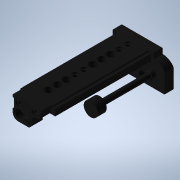
# Autodesk Inventor part: DGSL-12---(50-0-JP)
Saved by Autodesk Inventor 2021 (Build 250183000, 183)
## iProperties
Created: 2026-04-25
Part Number: DGSL-12---(50-0-JP)
Material: Generic
Catalog Web Link: www.3dfindit.com
Description: DGSL-(JP)-Plate
Vendor: FESTO
Document SubType Name: Modeling
Designer: psAdmin
Manufacturer: FESTO
Mass: 64.512 g
Surface Area: 242.987 cm^2
Volume: 64.512 cm^3
Density: 1 g/cm^3
Appearance: PSOLRGB-128-128-128
Category: PARTsolutions
Company: FESTO
Title: DGSL-12---(50-0-JP)
Author: Cadenas PARTsolutions
Comments: Plate
PSOL_IDENT_0: {$CADENAS_DATA/23d-libs/festo/parts/d/dgsl/parts/dgsl_jochplatten.prj},193 {VTYP=3D},{NB=DGSL-12---(
PSOL_IDENT_1: 50-0-JP)},{LINA=DGSL-12---(50-0-JP)},{NN=DGSL-(JP)},{DATE=08.01.2026 09:08:18},{GEOMDATE=08.01.2026
PSOL_IDENT_2: 09:08:00},{VERSION=},{LINEID=50},{WBVAR=DA,HUB},{WBNUMERIC=DA,HUB}  {NB=DGSL-12---(50-0-JP)},{LINA=D
PSOL_IDENT_3: GSL-12---(50-0-JP)},{KT=DUMMY},{TYP=DGSL-12},{KDM2=12},{DA=0},{HUB=50},{L1=108.6},{L1X=230.000},{SDD
PSOL_IDENT_4: N=10.000},{YOFF=0.000},{HUBW=[10:200]},{L2=10.000},{L4=50.000},{L9=10.000},{L15=5.800},{B4=24.000},{
PSOL_IDENT_5: B5=10.000},{BM=23.500},{H2=34.800},{H11=10.000},{H12=17.700},{KDM=16},{DIMBOHR=23.500},{DIMBOHRY=-15
PSOL_IDENT_6: .800},{KORRB4=0.200},{KORRH12=0.000},{A=1.750}
NB: DGSL-12---(50-0-JP)
NN: DGSL-(JP)
NT: Plate
NBSYN: $TYP.---($HUB.-$DA.-JP)
LINA: DGSL-12---(50-0-JP)
CATALOG: Festo
TYP: DGSL-12
KDM2: 12
DA: 0
HUB: 50
YOFF: 0
HUBW: [10:200]
L2: 10
L4: 50
L9: 10
L15: 5.8
B4: 24
B5: 10
BM: 23.5
H2: 34.8
H11: 10
H12: 17.7
KDM: 16
DIMBOHR: 23.5
DIMBOHRY: -15.8
KORRB4: 0.2
KORRH12: 0
A: 1.75
SUPPLIER: FESTO
ARTICLENO: DGSL-12---(50-0-JP)
BOMINFO: DGSL-12---(50-0-JP)
CREATOR: CADENAS GmbH
Autodesk Inventor part; units mm, degrees
sketch "Skizze_Jochplatte" plane through (0, 0, 0) normal (0, 0, 1) x (1, 0, 0)
  line L0 (0, 34.3) -> (0, 0)
  line L1 (0, 0) -> (58.5, 0)
  arc A0 (58.5, 0) -> (59, 0.5) centre (58.5, 0.5) ccw
  line L2 (59, 0.5) -> (59, 21.9765)
  arc A1 (59, 21.9765) -> (58.814286, 22.556964) centre (58, 21.9765) ccw
  arc A2 (58.814286, 22.556964) -> (46.894118, 28.847116) centre (46.6, 13.85) ccw
  arc A3 (46.6, 29.147059) -> (46.894118, 28.847116) centre (46.9, 29.147059) ccw
  line L3 (46.6, 29.147059) -> (46.6, 34.3)
  arc A4 (46.6, 34.3) -> (46.1, 34.8) centre (46.1, 34.3) ccw
  line L4 (46.1, 34.8) -> (0.5, 34.8)
  arc A5 (0.5, 34.8) -> (0, 34.3) centre (0.5, 34.3) ccw
  constraints: 12 point on circle, 10 end point, 6 centre point
sketch "Skizze_Jochplatte outline for Extrusion1" plane through (0, 0, 0) normal (0, 0, 1) x (1, 0, 0)
  arc A0 (0.5, 34.8) -> (0, 34.3) centre (0.5, 34.3) ccw
  line L0 (46.1, 34.8) -> (0.5, 34.8)
  arc A1 (46.6, 34.3) -> (46.1, 34.8) centre (46.1, 34.3) ccw
  line L1 (46.6, 29.147059) -> (46.6, 34.3)
  arc A2 (46.894118, 28.847116) -> (46.6, 29.147059) centre (46.9, 29.147059) cw
  arc A3 (58.814286, 22.556964) -> (46.894118, 28.847116) centre (46.6, 13.85) ccw
  arc A4 (59, 21.9765) -> (58.814286, 22.556964) centre (58, 21.9765) ccw
  line L2 (59, 0.5) -> (59, 21.9765)
  arc A5 (58.5, 0) -> (59, 0.5) centre (58.5, 0.5) ccw
  line L3 (0, 0) -> (58.5, 0)
  line L4 (0, 34.3) -> (0, 0)
extrude "Extrusion1" add sketch "Skizze_Jochplatte outline for Extrusion1" along normal blind 10
sketch "Sketch2" plane through (0, 0, 0) normal (0, 0, -1) x (-1, 0, 0)
  point P0 (-13.5, 7.1)
hole "Hole1" at (13.5, 7.1, 0) direction (0, 0, 1) diameter 7.8 depth 10 counterbore diameter 8 counterbore depth 7.5
sketch "Sketch3" plane through (0, 0, 0) normal (0, 0, -1) x (-1, 0, 0)
  point P0 (-33.5, 7.1)
hole "Hole2" at (33.5, 7.1, 0) direction (0, 0, 1) diameter 7.8 depth 10 counterbore diameter 8 counterbore depth 7.5
sketch "Skizze_JP_Bohrung_1C" plane through (0, 7.1, 0) normal (0, 1, 0) x (1, 0, 0)
  line L0 (23.5, -10) -> (23.5, 0)
  line L1 (23.5, 0) -> (27, 0)
  line L2 (27, 0) -> (27, -1.6)
  line L3 (27, -1.6) -> (26, -1.6)
  line L4 (26, -1.6) -> (25.567, -2.033)
  line L5 (25.567, -2.033) -> (25.567, -9.567)
  line L6 (25.567, -9.567) -> (26, -10)
  line L7 (26, -10) -> (23.5, -10)
  line L8 (23.5, -10) -> (23.5, 0)
  constraints: 18 end point
sketch "Skizze_JP_Bohrung_1C outline for Revolution1" plane through (0, 7.1, 0) normal (0, 1, 0) x (1, 0, 0)
  line L0 (23.5, 0) -> (27, 0)
  line L1 (27, 0) -> (27, -1.6)
  line L2 (27, -1.6) -> (26, -1.6)
  line L3 (26, -1.6) -> (25.567, -2.033)
  line L4 (25.567, -2.033) -> (25.567, -9.567)
  line L5 (25.567, -9.567) -> (26, -10)
  line L6 (26, -10) -> (23.5, -10)
  line L7 (23.5, -10) -> (23.5, 0)
revolve "Revolution1" cut sketch "Skizze_JP_Bohrung_1C outline for Revolution1" angle 360 about axis through (23.5, 7.1, 10) along (0, 0, 1)
thread "Thread1" size "M5x0.8" class "6H" standard "ISO Metric profile" full length
sketch "Skizze_JP_Bohrung_2A" plane through (0, 17.1, 0) normal (0, 1, 0) x (1, 0, 0)
  line L0 (13.5, -10) -> (13.5, 0)
  line L1 (13.5, 0) -> (17, 0)
  line L2 (17, 0) -> (17, -1.6)
  line L3 (17, -1.6) -> (16, -1.6)
  line L4 (16, -1.6) -> (15.567, -2.033)
  line L5 (15.567, -2.033) -> (15.567, -9.567)
  line L6 (15.567, -9.567) -> (16, -10)
  line L7 (16, -10) -> (13.5, -10)
  line L8 (13.5, -10) -> (13.5, 0)
  constraints: 18 end point
sketch "Skizze_JP_Bohrung_2A outline for Revolution2" plane through (0, 17.1, 0) normal (0, 1, 0) x (1, 0, 0)
  line L0 (13.5, 0) -> (17, 0)
  line L1 (17, 0) -> (17, -1.6)
  line L2 (17, -1.6) -> (16, -1.6)
  line L3 (16, -1.6) -> (15.567, -2.033)
  line L4 (15.567, -2.033) -> (15.567, -9.567)
  line L5 (15.567, -9.567) -> (16, -10)
  line L6 (16, -10) -> (13.5, -10)
  line L7 (13.5, -10) -> (13.5, 0)
revolve "Revolution2" cut sketch "Skizze_JP_Bohrung_2A outline for Revolution2" angle 360 about axis through (13.5, 17.1, 10) along (0, 0, 1)
thread "Thread2" size "M5x0.8" class "6H" standard "ISO Metric profile" full length
sketch "Skizze_JP_Bohrung_2B" plane through (0, 17.1, 0) normal (0, 1, 0) x (1, 0, 0)
  line L0 (23.5, -10) -> (23.5, 0)
  line L1 (23.5, 0) -> (27, 0)
  line L2 (27, 0) -> (27, -1.6)
  line L3 (27, -1.6) -> (26, -1.6)
  line L4 (26, -1.6) -> (25.567, -2.033)
  line L5 (25.567, -2.033) -> (25.567, -9.567)
  line L6 (25.567, -9.567) -> (26, -10)
  line L7 (26, -10) -> (23.5, -10)
  line L8 (23.5, -10) -> (23.5, 0)
  constraints: 18 end point
sketch "Skizze_JP_Bohrung_2B outline for Revolution3" plane through (0, 17.1, 0) normal (0, 1, 0) x (1, 0, 0)
  line L0 (23.5, 0) -> (27, 0)
  line L1 (27, 0) -> (27, -1.6)
  line L2 (27, -1.6) -> (26, -1.6)
  line L3 (26, -1.6) -> (25.567, -2.033)
  line L4 (25.567, -2.033) -> (25.567, -9.567)
  line L5 (25.567, -9.567) -> (26, -10)
  line L6 (26, -10) -> (23.5, -10)
  line L7 (23.5, -10) -> (23.5, 0)
revolve "Revolution3" cut sketch "Skizze_JP_Bohrung_2B outline for Revolution3" angle 360 about axis through (23.5, 17.1, 10) along (0, 0, 1)
thread "Thread3" size "M5x0.8" class "6H" standard "ISO Metric profile" full length
sketch "Skizze_JP_Bohrung_2C" plane through (0, 17.1, 0) normal (0, 1, 0) x (1, 0, 0)
  line L0 (33.5, -10) -> (33.5, 0)
  line L1 (33.5, 0) -> (37, 0)
  line L2 (37, 0) -> (37, -1.6)
  line L3 (37, -1.6) -> (36, -1.6)
  line L4 (36, -1.6) -> (35.567, -2.033)
  line L5 (35.567, -2.033) -> (35.567, -9.567)
  line L6 (35.567, -9.567) -> (36, -10)
  line L7 (36, -10) -> (33.5, -10)
  line L8 (33.5, -10) -> (33.5, 0)
  constraints: 18 end point
sketch "Skizze_JP_Bohrung_2C outline for Revolution4" plane through (0, 17.1, 0) normal (0, 1, 0) x (1, 0, 0)
  line L0 (33.5, 0) -> (37, 0)
  line L1 (37, 0) -> (37, -1.6)
  line L2 (37, -1.6) -> (36, -1.6)
  line L3 (36, -1.6) -> (35.567, -2.033)
  line L4 (35.567, -2.033) -> (35.567, -9.567)
  line L5 (35.567, -9.567) -> (36, -10)
  line L6 (36, -10) -> (33.5, -10)
  line L7 (33.5, -10) -> (33.5, 0)
revolve "Revolution4" cut sketch "Skizze_JP_Bohrung_2C outline for Revolution4" angle 360 about axis through (33.5, 17.1, 10) along (0, 0, 1)
thread "Thread4" size "M5x0.8" class "6H" standard "ISO Metric profile" full length
sketch "Skizze_JP_Bohrung_3" plane through (0, 27.1, 0) normal (0, 1, 0) x (1, 0, 0)
  line L0 (23.5, -10) -> (23.5, 0)
  line L1 (23.5, 0) -> (27, 0)
  line L2 (27, 0) -> (27, -1.6)
  line L3 (27, -1.6) -> (26, -1.6)
  line L4 (26, -1.6) -> (25.567, -2.033)
  line L5 (25.567, -2.033) -> (25.567, -9.567)
  line L6 (25.567, -9.567) -> (26, -10)
  line L7 (26, -10) -> (23.5, -10)
  line L8 (23.5, -10) -> (23.5, 0)
  constraints: 18 end point
sketch "Skizze_JP_Bohrung_3 outline for Revolution5" plane through (0, 27.1, 0) normal (0, 1, 0) x (1, 0, 0)
  line L0 (23.5, 0) -> (27, 0)
  line L1 (27, 0) -> (27, -1.6)
  line L2 (27, -1.6) -> (26, -1.6)
  line L3 (26, -1.6) -> (25.567, -2.033)
  line L4 (25.567, -2.033) -> (25.567, -9.567)
  line L5 (25.567, -9.567) -> (26, -10)
  line L6 (26, -10) -> (23.5, -10)
  line L7 (23.5, -10) -> (23.5, 0)
revolve "Revolution5" cut sketch "Skizze_JP_Bohrung_3 outline for Revolution5" angle 360 about axis through (23.5, 27.1, 10) along (0, 0, 1)
thread "Thread5" size "M5x0.8" class "6H" standard "ISO Metric profile" full length
sketch "Sketch_2" plane through (0, 29.6, 0) normal (0, 1, 0) x (1, 0, 0)
  line L0 (14.5, -4.6) -> (14.5, 0)
  line L1 (14.5, 0) -> (18.5, 0)
  line L2 (18.5, 0) -> (18.5, -4.6)
  line L3 (18.5, -4.6) -> (18.45, -4.6)
  line L4 (18.45, -4.6) -> (18.45, -1)
  arc A0 (18.45, -1) -> (18.05, -0.6) centre (18.05, -1) ccw
  line L5 (18.05, -0.6) -> (14.5, -0.6)
  line L6 (14.5, -0.6) -> (14.5, 0)
  constraints: 14 end point, 2 point on circle, 1 centre point
sketch "Sketch_2 outline for Revolution6" plane through (0, 29.6, 0) normal (0, 1, 0) x (1, 0, 0)
  line L0 (14.5, 0) -> (18.5, 0)
  line L1 (18.5, 0) -> (18.5, -4.6)
  line L2 (18.5, -4.6) -> (18.45, -4.6)
  line L3 (18.45, -4.6) -> (18.45, -1)
  arc A0 (18.45, -1) -> (18.05, -0.6) centre (18.05, -1) ccw
  line L4 (18.05, -0.6) -> (14.5, -0.6)
  line L5 (14.5, -0.6) -> (14.5, 0)
revolve "Revolution6" cut sketch "Sketch_2 outline for Revolution6" angle 360 about axis through (14.5, 29.6, 4.6) along (0, 0, 1)
sketch "Sketch_8" plane through (0, 29.6, 0) normal (0, 1, 0) x (1, 0, 0)
  line L0 (32.5, -4.6) -> (32.5, 0)
  line L1 (32.5, 0) -> (36.5, 0)
  line L2 (36.5, 0) -> (36.5, -4.6)
  line L3 (36.5, -4.6) -> (36.45, -4.6)
  line L4 (36.45, -4.6) -> (36.45, -1)
  arc A0 (36.45, -1) -> (36.05, -0.6) centre (36.05, -1) ccw
  line L5 (36.05, -0.6) -> (32.5, -0.6)
  line L6 (32.5, -0.6) -> (32.5, 0)
  constraints: 14 end point, 2 point on circle, 1 centre point
sketch "Sketch_8 outline for Revolution7" plane through (0, 29.6, 0) normal (0, 1, 0) x (1, 0, 0)
  line L0 (32.5, 0) -> (36.5, 0)
  line L1 (36.5, 0) -> (36.5, -4.6)
  line L2 (36.5, -4.6) -> (36.45, -4.6)
  line L3 (36.45, -4.6) -> (36.45, -1)
  arc A0 (36.45, -1) -> (36.05, -0.6) centre (36.05, -1) ccw
  line L4 (36.05, -0.6) -> (32.5, -0.6)
  line L5 (32.5, -0.6) -> (32.5, 0)
revolve "Revolution7" cut sketch "Sketch_8 outline for Revolution7" angle 360 about axis through (32.5, 29.6, 4.6) along (0, 0, 1)
sketch "Sketch_7" plane through (14.5, 29.6, 0.6) normal (0, 0, -1) x (1, 0, 0)
  line L0 (-1.5, -0.866025) -> (0, -1.732051)
  line L1 (0, -1.732051) -> (1.5, -0.866025)
  line L2 (1.5, -0.866025) -> (1.5, 0.866025)
  line L3 (1.5, 0.866025) -> (0, 1.732051)
  line L4 (0, 1.732051) -> (-1.5, 0.866025)
  line L5 (-1.5, 0.866025) -> (-1.5, -0.866025)
  constraints: 12 end point
sketch "Sketch_7 outline for Extrusion2" plane through (14.5, 29.6, 0.6) normal (0, 0, -1) x (1, 0, 0)
  line L0 (-1.5, 0.866025) -> (-1.5, -0.866025)
  line L1 (0, 1.732051) -> (-1.5, 0.866025)
  line L2 (1.5, 0.866025) -> (0, 1.732051)
  line L3 (1.5, -0.866025) -> (1.5, 0.866025)
  line L4 (0, -1.732051) -> (1.5, -0.866025)
  line L5 (-1.5, -0.866025) -> (0, -1.732051)
extrude "Extrusion2" cut sketch "Sketch_7 outline for Extrusion2" against normal blind 2.2
sketch "Sketch_15" plane through (32.5, 29.6, 0.6) normal (0, 0, -1) x (1, 0, 0)
  line L0 (-1.5, -0.866025) -> (0, -1.732051)
  line L1 (0, -1.732051) -> (1.5, -0.866025)
  line L2 (1.5, -0.866025) -> (1.5, 0.866025)
  line L3 (1.5, 0.866025) -> (0, 1.732051)
  line L4 (0, 1.732051) -> (-1.5, 0.866025)
  line L5 (-1.5, 0.866025) -> (-1.5, -0.866025)
  constraints: 12 end point
sketch "Sketch_15 outline for Extrusion3" plane through (32.5, 29.6, 0.6) normal (0, 0, -1) x (1, 0, 0)
  line L0 (-1.5, 0.866025) -> (-1.5, -0.866025)
  line L1 (0, 1.732051) -> (-1.5, 0.866025)
  line L2 (1.5, 0.866025) -> (0, 1.732051)
  line L3 (1.5, -0.866025) -> (1.5, 0.866025)
  line L4 (0, -1.732051) -> (1.5, -0.866025)
  line L5 (-1.5, -0.866025) -> (0, -1.732051)
extrude "Extrusion3" cut sketch "Sketch_15 outline for Extrusion3" against normal blind 2.2
sketch "Skizze_JP_Bohrung_5" plane through (0, 13.8, 0) normal (0, 1, 0) x (1, 0, 0)
  line L0 (45.1, -4.6) -> (45.1, 0)
  line L1 (45.1, 0) -> (49.1, 0)
  line L2 (49.1, 0) -> (49.1, -4.6)
  line L3 (49.1, -4.6) -> (48.6, -4.6)
  line L4 (48.6, -4.6) -> (48.6, -1)
  arc A0 (48.6, -1) -> (48.2, -0.6) centre (48.2, -1) ccw
  line L5 (48.2, -0.6) -> (46.842, -0.6)
  line L6 (46.842, -0.6) -> (45.1, -1.234036)
  line L7 (45.1, -1.234036) -> (45.1, 0)
  constraints: 16 end point, 2 point on circle, 1 centre point
sketch "Skizze_JP_Bohrung_5 outline for Revolution8" plane through (0, 13.8, 0) normal (0, 1, 0) x (1, 0, 0)
  line L0 (45.1, 0) -> (49.1, 0)
  line L1 (49.1, 0) -> (49.1, -4.6)
  line L2 (49.1, -4.6) -> (48.6, -4.6)
  line L3 (48.6, -4.6) -> (48.6, -1)
  arc A0 (48.6, -1) -> (48.2, -0.6) centre (48.2, -1) ccw
  line L4 (48.2, -0.6) -> (46.842, -0.6)
  line L5 (46.842, -0.6) -> (45.1, -1.234036)
  line L6 (45.1, -1.234036) -> (45.1, 0)
revolve "Revolution8" cut sketch "Skizze_JP_Bohrung_5 outline for Revolution8" angle 360 about axis through (45.1, 13.8, 4.6) along (0, 0, 1)
sketch "Skizze_JP_Bohrung_5_HEX" plane through (45.1, 13.8, 0.6) normal (0, 0, -1) x (1, 0, 0)
  line L0 (-1.5, -0.866025) -> (0, -1.732051)
  line L1 (0, -1.732051) -> (1.5, -0.866025)
  line L2 (1.5, -0.866025) -> (1.5, 0.866025)
  line L3 (1.5, 0.866025) -> (0, 1.732051)
  line L4 (0, 1.732051) -> (-1.5, 0.866025)
  line L5 (-1.5, 0.866025) -> (-1.5, -0.866025)
  constraints: 12 end point
sketch "Skizze_JP_Bohrung_5_HEX outline for Extrusion4" plane through (45.1, 13.8, 0.6) normal (0, 0, -1) x (1, 0, 0)
  line L0 (-1.5, 0.866025) -> (-1.5, -0.866025)
  line L1 (0, 1.732051) -> (-1.5, 0.866025)
  line L2 (1.5, 0.866025) -> (0, 1.732051)
  line L3 (1.5, -0.866025) -> (1.5, 0.866025)
  line L4 (0, -1.732051) -> (1.5, -0.866025)
  line L5 (-1.5, -0.866025) -> (0, -1.732051)
extrude "Extrusion4" cut sketch "Skizze_JP_Bohrung_5_HEX outline for Extrusion4" against normal blind 2
sketch "Sketch_6" plane through (0, 13.8, 0) normal (0, 1, 0) x (1, 0, 0)
  line L0 (45.1, -80) -> (45.1, -10)
  line L1 (45.1, -10) -> (49.14, -10)
  line L2 (49.14, -10) -> (49.14, -14.15)
  line L3 (49.14, -14.15) -> (48.84, -14.45)
  line L4 (48.84, -14.45) -> (48.1, -14.45)
  line L5 (48.1, -14.45) -> (48.1, -70)
  line L6 (48.1, -70) -> (53.1, -70)
  line L7 (53.1, -70) -> (53.1, -80)
  line L8 (53.1, -80) -> (45.1, -80)
  line L9 (45.1, -80) -> (45.1, -10)
  constraints: 20 end point
sketch "Sketch_6 outline for Revolution9" plane through (0, 13.8, 0) normal (0, 1, 0) x (1, 0, 0)
  line L0 (45.1, -10) -> (49.14, -10)
  line L1 (49.14, -10) -> (49.14, -14.15)
  line L2 (49.14, -14.15) -> (48.84, -14.45)
  line L3 (48.84, -14.45) -> (48.1, -14.45)
  line L4 (48.1, -14.45) -> (48.1, -70)
  line L5 (48.1, -70) -> (53.1, -70)
  line L6 (53.1, -70) -> (53.1, -80)
  line L7 (53.1, -80) -> (45.1, -80)
  line L8 (45.1, -80) -> (45.1, -10)
revolve "Revolution9" add sketch "Sketch_6 outline for Revolution9" angle 360 about axis through (45.1, 13.8, 80) along (0, 0, 1)
sketch "Skizze_Schiene" plane through (0, 0, 10) normal (0, 0, 1) x (1, 0, 0)
  arc A0 (3.55, 25.3) -> (3.75, 25.1) centre (3.75, 25.3) ccw
  line L0 (3.75, 25.1) -> (11, 25.1)
  line L1 (11, 25.1) -> (11, 25)
  line L2 (11, 25) -> (36, 25)
  line L3 (36, 25) -> (36, 25.1)
  line L4 (36, 25.1) -> (43.25, 25.1)
  arc A1 (43.25, 25.1) -> (43.45, 25.3) centre (43.25, 25.3) ccw
  line L5 (43.45, 25.3) -> (43.45, 32.5)
  line L6 (43.45, 32.5) -> (40.5, 32.5)
  line L7 (40.5, 32.5) -> (40.5, 34.15359)
  line L8 (40.5, 34.15359) -> (41.1, 34.5)
  line L9 (41.1, 34.5) -> (41.1, 35)
  line L10 (41.1, 35) -> (5.9, 35)
  line L11 (5.9, 35) -> (5.9, 34.5)
  line L12 (5.9, 34.5) -> (6.5, 34.15359)
  line L13 (6.5, 34.15359) -> (6.5, 32.5)
  line L14 (6.5, 32.5) -> (3.55, 32.5)
  line L15 (3.55, 32.5) -> (3.55, 25.3)
  constraints: 32 end point, 4 point on circle, 2 centre point
sketch "Skizze_Schiene outline for Extrusion5" plane through (0, 0, 10) normal (0, 0, 1) x (1, 0, 0)
  line L0 (3.55, 32.5) -> (3.55, 25.3)
  line L1 (6.5, 32.5) -> (3.55, 32.5)
  line L2 (6.5, 34.15359) -> (6.5, 32.5)
  line L3 (5.9, 34.5) -> (6.5, 34.15359)
  line L4 (5.9, 35) -> (5.9, 34.5)
  line L5 (41.1, 35) -> (5.9, 35)
  line L6 (41.1, 34.5) -> (41.1, 35)
  line L7 (40.5, 34.15359) -> (41.1, 34.5)
  line L8 (40.5, 32.5) -> (40.5, 34.15359)
  line L9 (43.45, 32.5) -> (40.5, 32.5)
  line L10 (43.45, 25.3) -> (43.45, 32.5)
  arc A0 (43.25, 25.1) -> (43.45, 25.3) centre (43.25, 25.3) ccw
  line L11 (36, 25.1) -> (43.25, 25.1)
  line L12 (36, 25) -> (36, 25.1)
  line L13 (11, 25) -> (36, 25)
  line L14 (11, 25.1) -> (11, 25)
  line L15 (3.75, 25.1) -> (11, 25.1)
  arc A1 (3.55, 25.3) -> (3.75, 25.1) centre (3.75, 25.3) ccw
extrude "Extrusion5" add sketch "Skizze_Schiene outline for Extrusion5" along normal blind 108.6
sketch "Skizze_Endplatte" plane through (0, 0, 118.6) normal (0, 0, 1) x (1, 0, 0)
  line L0 (7.1, 32.65) -> (8.45, 31.3)
  line L1 (8.45, 31.3) -> (8.45, 22.5)
  line L2 (8.45, 22.5) -> (7.1, 21.15)
  line L3 (7.1, 21.15) -> (7.1, 17.2)
  arc A0 (7.1, 17.2) -> (13.1, 11.2) centre (13.1, 17.2) ccw
  line L4 (13.1, 11.2) -> (25.7, 11.2)
  line L5 (25.7, 11.2) -> (29.2, 14.7)
  line L6 (29.2, 14.7) -> (29.2, 21.5)
  arc A1 (32.2, 24.5) -> (29.2, 21.5) centre (32.2, 21.5) ccw
  line L7 (32.2, 24.5) -> (36.55, 24.5)
  line L8 (36.55, 24.5) -> (38.55, 26.5)
  line L9 (38.55, 26.5) -> (38.55, 31.3)
  line L10 (38.55, 31.3) -> (39.9, 32.65)
  line L11 (39.9, 32.65) -> (39.9, 34.8)
  line L12 (39.9, 34.8) -> (7.1, 34.8)
  line L13 (7.1, 34.8) -> (7.1, 32.65)
  constraints: 28 end point, 4 point on circle, 2 centre point
sketch "Skizze_Endplatte outline for Extrusion6" plane through (0, 0, 118.6) normal (0, 0, 1) x (1, 0, 0)
  line L0 (7.1, 34.8) -> (7.1, 32.65)
  line L1 (39.9, 34.8) -> (7.1, 34.8)
  line L2 (39.9, 32.65) -> (39.9, 34.8)
  line L3 (38.55, 31.3) -> (39.9, 32.65)
  line L4 (38.55, 26.5) -> (38.55, 31.3)
  line L5 (36.55, 24.5) -> (38.55, 26.5)
  line L6 (32.2, 24.5) -> (36.55, 24.5)
  arc A0 (29.2, 21.5) -> (32.2, 24.5) centre (32.2, 21.5) cw
  line L7 (29.2, 14.7) -> (29.2, 21.5)
  line L8 (25.7, 11.2) -> (29.2, 14.7)
  line L9 (13.1, 11.2) -> (25.7, 11.2)
  arc A1 (7.1, 17.2) -> (13.1, 11.2) centre (13.1, 17.2) ccw
  line L10 (7.1, 21.15) -> (7.1, 17.2)
  line L11 (8.45, 22.5) -> (7.1, 21.15)
  line L12 (8.45, 31.3) -> (8.45, 22.5)
  line L13 (7.1, 32.65) -> (8.45, 31.3)
extrude "Extrusion6" add sketch "Skizze_Endplatte outline for Extrusion6" along normal blind 12
sketch "Sketch_11" plane through (0, 29.6, 0) normal (0, 1, 0) x (1, 0, 0)
  line L0 (14.5, -130.6) -> (14.5, -126)
  line L1 (14.5, -130) -> (17.6, -130)
  arc A0 (17.6, -130) -> (18, -129.6) centre (17.6, -129.6) ccw
  line L2 (18, -129.6) -> (18, -126)
  line L3 (18, -126) -> (18.5, -126)
  line L4 (18.5, -126) -> (18.5, -130.6)
  line L5 (18.5, -130.6) -> (14.5, -130.6)
  line L6 (14.5, -130.6) -> (14.5, -130)
  constraints: 14 end point, 2 point on circle, 1 centre point
sketch "Sketch_11 outline for Revolution10" plane through (0, 29.6, 0) normal (0, 1, 0) x (1, 0, 0)
  line L0 (14.5, -130) -> (17.6, -130)
  arc A0 (17.6, -130) -> (18, -129.6) centre (17.6, -129.6) ccw
  line L1 (18, -129.6) -> (18, -126)
  line L2 (18, -126) -> (18.5, -126)
  line L3 (18.5, -126) -> (18.5, -130.6)
  line L4 (18.5, -130.6) -> (14.5, -130.6)
  line L5 (14.5, -130.6) -> (14.5, -130)
revolve "Revolution10" cut sketch "Sketch_11 outline for Revolution10" angle 360 about axis through (14.5, 29.6, 130.6) along (0, 0, 1)
sketch "Sketch_12" plane through (0, 29.6, 0) normal (0, 1, 0) x (1, 0, 0)
  line L0 (32.5, -130.6) -> (32.5, -126)
  line L1 (32.5, -130) -> (35.6, -130)
  arc A0 (35.6, -130) -> (36, -129.6) centre (35.6, -129.6) ccw
  line L2 (36, -129.6) -> (36, -126)
  line L3 (36, -126) -> (36.5, -126)
  line L4 (36.5, -126) -> (36.5, -130.6)
  line L5 (36.5, -130.6) -> (32.5, -130.6)
  line L6 (32.5, -130.6) -> (32.5, -130)
  constraints: 14 end point, 2 point on circle, 1 centre point
sketch "Sketch_12 outline for Revolution11" plane through (0, 29.6, 0) normal (0, 1, 0) x (1, 0, 0)
  line L0 (32.5, -130) -> (35.6, -130)
  arc A0 (35.6, -130) -> (36, -129.6) centre (35.6, -129.6) ccw
  line L1 (36, -129.6) -> (36, -126)
  line L2 (36, -126) -> (36.5, -126)
  line L3 (36.5, -126) -> (36.5, -130.6)
  line L4 (36.5, -130.6) -> (32.5, -130.6)
  line L5 (32.5, -130.6) -> (32.5, -130)
revolve "Revolution11" cut sketch "Sketch_12 outline for Revolution11" angle 360 about axis through (32.5, 29.6, 130.6) along (0, 0, 1)
sketch "Sketch_16" plane through (32.5, 29.6, 130) normal (0, 0, 1) x (1, 0, 0)
  line L0 (-1.732051, 0) -> (-0.866025, -1.5)
  line L1 (-0.866025, -1.5) -> (0.866025, -1.5)
  line L2 (0.866025, -1.5) -> (1.732051, 0)
  line L3 (1.732051, 0) -> (0.866025, 1.5)
  line L4 (0.866025, 1.5) -> (-0.866025, 1.5)
  line L5 (-0.866025, 1.5) -> (-1.732051, 0)
  constraints: 12 end point
sketch "Sketch_16 outline for Extrusion7" plane through (32.5, 29.6, 130) normal (0, 0, 1) x (1, 0, 0)
  line L0 (-0.866025, 1.5) -> (-1.732051, 0)
  line L1 (0.866025, 1.5) -> (-0.866025, 1.5)
  line L2 (1.732051, 0) -> (0.866025, 1.5)
  line L3 (0.866025, -1.5) -> (1.732051, 0)
  line L4 (-0.866025, -1.5) -> (0.866025, -1.5)
  line L5 (-1.732051, 0) -> (-0.866025, -1.5)
extrude "Extrusion7" cut sketch "Sketch_16 outline for Extrusion7" against normal blind 2
sketch "Sketch_17" plane through (14.5, 29.6, 130) normal (0, 0, 1) x (1, 0, 0)
  line L0 (-1.732051, 0) -> (-0.866025, -1.5)
  line L1 (-0.866025, -1.5) -> (0.866025, -1.5)
  line L2 (0.866025, -1.5) -> (1.732051, 0)
  line L3 (1.732051, 0) -> (0.866025, 1.5)
  line L4 (0.866025, 1.5) -> (-0.866025, 1.5)
  line L5 (-0.866025, 1.5) -> (-1.732051, 0)
  constraints: 12 end point
sketch "Sketch_17 outline for Extrusion8" plane through (14.5, 29.6, 130) normal (0, 0, 1) x (1, 0, 0)
  line L0 (-0.866025, 1.5) -> (-1.732051, 0)
  line L1 (0.866025, 1.5) -> (-0.866025, 1.5)
  line L2 (1.732051, 0) -> (0.866025, 1.5)
  line L3 (0.866025, -1.5) -> (1.732051, 0)
  line L4 (-0.866025, -1.5) -> (0.866025, -1.5)
  line L5 (-1.732051, 0) -> (-0.866025, -1.5)
extrude "Extrusion8" cut sketch "Sketch_17 outline for Extrusion8" against normal blind 2
sketch "Skizze_1" plane through (23.5, 0, 0) normal (1, 0, 0) x (0, 0, -1)
  line L0 (-15.8, 25) -> (-15.8, 35)
  line L1 (-15.8, 35) -> (-12.3, 35)
  line L2 (-12.3, 35) -> (-12.3, 33.4)
  line L3 (-12.3, 33.4) -> (-13.3, 33.4)
  line L4 (-13.3, 33.4) -> (-13.733, 32.967)
  line L5 (-13.733, 32.967) -> (-13.733, 25.433)
  line L6 (-13.733, 25.433) -> (-13.3, 25)
  line L7 (-13.3, 25) -> (-15.8, 25)
  line L8 (-15.8, 25) -> (-15.8, 35)
  constraints: 18 end point
sketch "Skizze_1 outline for Revolution12" plane through (23.5, 0, 0) normal (1, 0, 0) x (0, 0, -1)
  line L0 (-15.8, 35) -> (-12.3, 35)
  line L1 (-12.3, 35) -> (-12.3, 33.4)
  line L2 (-12.3, 33.4) -> (-13.3, 33.4)
  line L3 (-13.3, 33.4) -> (-13.733, 32.967)
  line L4 (-13.733, 32.967) -> (-13.733, 25.433)
  line L5 (-13.733, 25.433) -> (-13.3, 25)
  line L6 (-13.3, 25) -> (-15.8, 25)
  line L7 (-15.8, 25) -> (-15.8, 35)
revolve "Revolution12" cut sketch "Skizze_1 outline for Revolution12" angle 360 about axis through (23.5, 25, 15.8) along (0, -1, 0)
thread "Thread6" size "M5x0.8" class "6H" standard "ISO Metric profile" full length
sketch "Skizze_2" plane through (23.5, 0, 0) normal (1, 0, 0) x (0, 0, -1)
  line L0 (-25.8, 25) -> (-25.8, 35)
  line L1 (-25.8, 35) -> (-22.3, 35)
  line L2 (-22.3, 35) -> (-22.3, 33.4)
  line L3 (-22.3, 33.4) -> (-23.3, 33.4)
  line L4 (-23.3, 33.4) -> (-23.733, 32.967)
  line L5 (-23.733, 32.967) -> (-23.733, 25.433)
  line L6 (-23.733, 25.433) -> (-23.3, 25)
  line L7 (-23.3, 25) -> (-25.8, 25)
  line L8 (-25.8, 25) -> (-25.8, 35)
  constraints: 18 end point
sketch "Skizze_2 outline for Revolution13" plane through (23.5, 0, 0) normal (1, 0, 0) x (0, 0, -1)
  line L0 (-25.8, 35) -> (-22.3, 35)
  line L1 (-22.3, 35) -> (-22.3, 33.4)
  line L2 (-22.3, 33.4) -> (-23.3, 33.4)
  line L3 (-23.3, 33.4) -> (-23.733, 32.967)
  line L4 (-23.733, 32.967) -> (-23.733, 25.433)
  line L5 (-23.733, 25.433) -> (-23.3, 25)
  line L6 (-23.3, 25) -> (-25.8, 25)
  line L7 (-25.8, 25) -> (-25.8, 35)
revolve "Revolution13" cut sketch "Skizze_2 outline for Revolution13" angle 360 about axis through (23.5, 25, 25.8) along (0, -1, 0)
thread "Thread7" size "M5x0.8" class "6H" standard "ISO Metric profile" full length
sketch "Sketch24" plane through (22.143534, 25, 10) normal (0, -1, 0) x (1, 0, 0)
  point P0 (1.356466, 25.8)
hole "Hole3" at (23.5, 25, 35.8) direction (0, 1, 0) diameter 9 depth 10
sketch "Sketch25" plane through (22.143534, 25, 10) normal (0, -1, 0) x (1, 0, 0)
  point P0 (1.356466, 35.8)
hole "Hole4" at (23.5, 25, 45.8) direction (0, 1, 0) diameter 9 depth 10
sketch "Sketch26" plane through (22.143534, 25, 10) normal (0, -1, 0) x (1, 0, 0)
  point P0 (1.356466, 45.8)
hole "Hole5" at (23.5, 25, 55.8) direction (0, 1, 0) diameter 9 depth 10
sketch "Skizze_6" plane through (23.5, 0, 0) normal (1, 0, 0) x (0, 0, -1)
  line L0 (-65.8, 25) -> (-65.8, 35)
  line L1 (-65.8, 35) -> (-62.3, 35)
  line L2 (-62.3, 35) -> (-62.3, 33.4)
  line L3 (-62.3, 33.4) -> (-63.3, 33.4)
  line L4 (-63.3, 33.4) -> (-63.733, 32.967)
  line L5 (-63.733, 32.967) -> (-63.733, 25.433)
  line L6 (-63.733, 25.433) -> (-63.3, 25)
  line L7 (-63.3, 25) -> (-65.8, 25)
  line L8 (-65.8, 25) -> (-65.8, 35)
  constraints: 18 end point
sketch "Skizze_6 outline for Revolution14" plane through (23.5, 0, 0) normal (1, 0, 0) x (0, 0, -1)
  line L0 (-65.8, 35) -> (-62.3, 35)
  line L1 (-62.3, 35) -> (-62.3, 33.4)
  line L2 (-62.3, 33.4) -> (-63.3, 33.4)
  line L3 (-63.3, 33.4) -> (-63.733, 32.967)
  line L4 (-63.733, 32.967) -> (-63.733, 25.433)
  line L5 (-63.733, 25.433) -> (-63.3, 25)
  line L6 (-63.3, 25) -> (-65.8, 25)
  line L7 (-65.8, 25) -> (-65.8, 35)
revolve "Revolution14" cut sketch "Skizze_6 outline for Revolution14" angle 360 about axis through (23.5, 25, 65.8) along (0, -1, 0)
thread "Thread8" size "M5x0.8" class "6H" standard "ISO Metric profile" full length
sketch "Skizze_7" plane through (23.5, 0, 0) normal (1, 0, 0) x (0, 0, -1)
  line L0 (-75.8, 25) -> (-75.8, 35)
  line L1 (-75.8, 35) -> (-72.3, 35)
  line L2 (-72.3, 35) -> (-72.3, 33.4)
  line L3 (-72.3, 33.4) -> (-73.3, 33.4)
  line L4 (-73.3, 33.4) -> (-73.733, 32.967)
  line L5 (-73.733, 32.967) -> (-73.733, 25.433)
  line L6 (-73.733, 25.433) -> (-73.3, 25)
  line L7 (-73.3, 25) -> (-75.8, 25)
  line L8 (-75.8, 25) -> (-75.8, 35)
  constraints: 18 end point
sketch "Skizze_7 outline for Revolution15" plane through (23.5, 0, 0) normal (1, 0, 0) x (0, 0, -1)
  line L0 (-75.8, 35) -> (-72.3, 35)
  line L1 (-72.3, 35) -> (-72.3, 33.4)
  line L2 (-72.3, 33.4) -> (-73.3, 33.4)
  line L3 (-73.3, 33.4) -> (-73.733, 32.967)
  line L4 (-73.733, 32.967) -> (-73.733, 25.433)
  line L5 (-73.733, 25.433) -> (-73.3, 25)
  line L6 (-73.3, 25) -> (-75.8, 25)
  line L7 (-75.8, 25) -> (-75.8, 35)
revolve "Revolution15" cut sketch "Skizze_7 outline for Revolution15" angle 360 about axis through (23.5, 25, 75.8) along (0, -1, 0)
thread "Thread9" size "M5x0.8" class "6H" standard "ISO Metric profile" full length
sketch "Sketch29" plane through (22.143534, 25, 10) normal (0, -1, 0) x (1, 0, 0)
  point P0 (1.356466, 75.8)
hole "Hole6" at (23.5, 25, 85.8) direction (0, 1, 0) diameter 9 depth 10
sketch "Sketch30" plane through (22.143534, 25, 10) normal (0, -1, 0) x (1, 0, 0)
  point P0 (1.356466, 85.8)
hole "Hole7" at (23.5, 25, 95.8) direction (0, 1, 0) diameter 9 depth 10
sketch "Sketch31" plane through (22.143534, 25, 10) normal (0, -1, 0) x (1, 0, 0)
  point P0 (1.356466, 95.8)
hole "Hole8" at (23.5, 25, 105.8) direction (0, 1, 0) diameter 9 depth 10
sketch "Sketch_1" plane through (0, 0, 130.6) normal (0, 0, 1) x (1, 0, 0)
  arc A0 (16.171869, 22.572497) -> (14.59167, 13.610747) centre (15.381769, 18.091622) ccw
  line L0 (14.59167, 13.610747) -> (22.470132, 12.221561)
  arc A1 (22.470132, 12.221561) -> (24.050331, 21.183312) centre (23.260231, 16.702437) ccw
  line L1 (24.050331, 21.183312) -> (16.171869, 22.572497)
  constraints: 4 end point, 4 point on circle, 2 centre point
sketch "Sketch_1 outline for Extrusion9" plane through (0, 0, 130.6) normal (0, 0, 1) x (1, 0, 0)
  line L0 (24.050331, 21.183312) -> (16.171869, 22.572497)
  arc A0 (22.470132, 12.221561) -> (24.050331, 21.183312) centre (23.260231, 16.702437) ccw
  line L1 (14.59167, 13.610747) -> (22.470132, 12.221561)
  arc A1 (16.171869, 22.572497) -> (14.59167, 13.610747) centre (15.381769, 18.091622) ccw
extrude "Extrusion9" cut sketch "Sketch_1 outline for Extrusion9" against normal blind 5.5
sketch "Sketch_5" plane through (0, 0, 125.1) normal (0, 0, 1) x (1, 0, 0)
  line L0 (16.433261, 13.286025) -> (22.470132, 12.221561)
  arc A0 (22.470132, 12.221561) -> (24.050331, 21.183312) centre (23.260231, 16.702437) ccw
  line L1 (24.050331, 21.183312) -> (18.013459, 22.247775)
  line L2 (18.013459, 22.247775) -> (16.433261, 13.286025)
  constraints: 6 end point, 2 point on circle, 1 centre point
sketch "Sketch_5 outline for Extrusion10" plane through (0, 0, 125.1) normal (0, 0, 1) x (1, 0, 0)
  line L0 (18.013459, 22.247775) -> (16.433261, 13.286025)
  line L1 (24.050331, 21.183312) -> (18.013459, 22.247775)
  arc A0 (22.470132, 12.221561) -> (24.050331, 21.183312) centre (23.260231, 16.702437) ccw
  line L2 (16.433261, 13.286025) -> (22.470132, 12.221561)
extrude "Extrusion10" add sketch "Sketch_5 outline for Extrusion10" along normal blind 4.5
sketch "Skizze_Endplatte_Stossdaempfer_Bohrung" plane through (14.2, 0, 0) normal (1, 0, 0) x (0, 0, -1)
  line L0 (-118.6, 18.3) -> (-130.6, 18.3)
  line L1 (-130.6, 18.3) -> (-130.6, 23.45132)
  line L2 (-130.6, 23.45132) -> (-130.2, 22.7585)
  line L3 (-130.2, 22.7585) -> (-119, 22.7585)
  line L4 (-119, 22.7585) -> (-118.6, 23.45132)
  line L5 (-118.6, 23.45132) -> (-118.6, 18.3)
  line L6 (-118.6, 18.3) -> (-130.6, 18.3)
  constraints: 14 end point
sketch "Skizze_Endplatte_Stossdaempfer_Bohrung outline for Revolution16" plane through (14.2, 0, 0) normal (1, 0, 0) x (0, 0, -1)
  line L0 (-130.6, 18.3) -> (-130.6, 23.45132)
  line L1 (-130.6, 23.45132) -> (-130.2, 22.7585)
  line L2 (-130.2, 22.7585) -> (-119, 22.7585)
  line L3 (-119, 22.7585) -> (-118.6, 23.45132)
  line L4 (-118.6, 23.45132) -> (-118.6, 18.3)
  line L5 (-118.6, 18.3) -> (-130.6, 18.3)
revolve "Revolution16" cut sketch "Skizze_Endplatte_Stossdaempfer_Bohrung outline for Revolution16" angle 360 about axis through (14.2, 18.3, 118.6) along (0, 0, -1)
thread "Thread10" size "M10x1" class "6H" standard "ISO Metric profile" full length
sketch "Sketch_4" plane through (23.260231, 0, 0) normal (1, 0, 0) x (0, 0, -1)
  line L0 (-130.6, 16.702437) -> (-125.6, 16.702437)
  line L1 (-125.6, 16.702437) -> (-125.6, 13.702437)
  line L2 (-125.6, 13.702437) -> (-130, 13.702437)
  line L3 (-130, 13.702437) -> (-130.6, 14.302437)
  line L4 (-130.6, 14.302437) -> (-130.6, 16.702437)
  line L5 (-130.6, 16.702437) -> (-125.6, 16.702437)
  constraints: 12 end point
sketch "Sketch_4 outline for Revolution17" plane through (23.260231, 0, 0) normal (1, 0, 0) x (0, 0, -1)
  line L0 (-125.6, 16.702437) -> (-125.6, 13.702437)
  line L1 (-125.6, 13.702437) -> (-130, 13.702437)
  line L2 (-130, 13.702437) -> (-130.6, 14.302437)
  line L3 (-130.6, 14.302437) -> (-130.6, 16.702437)
  line L4 (-130.6, 16.702437) -> (-125.6, 16.702437)
revolve "Revolution17" add sketch "Sketch_4 outline for Revolution17" angle 360 about axis through (23.260231, 16.702437, 130.6) along (0, 0, 1)
sketch "Sketch_3" plane through (0, 0, 130.6) normal (0, 0, 1) x (1, 0, 0)
  line L0 (21.760231, 15.836411) -> (23.260231, 14.970386)
  line L1 (23.260231, 14.970386) -> (24.760231, 15.836411)
  line L2 (24.760231, 15.836411) -> (24.760231, 17.568462)
  line L3 (24.760231, 17.568462) -> (23.260231, 18.434488)
  line L4 (23.260231, 18.434488) -> (21.760231, 17.568462)
  line L5 (21.760231, 17.568462) -> (21.760231, 15.836411)
  constraints: 12 end point
sketch "Sketch_3 outline for Extrusion11" plane through (0, 0, 130.6) normal (0, 0, 1) x (1, 0, 0)
  line L0 (21.760231, 17.568462) -> (21.760231, 15.836411)
  line L1 (23.260231, 18.434488) -> (21.760231, 17.568462)
  line L2 (24.760231, 17.568462) -> (23.260231, 18.434488)
  line L3 (24.760231, 15.836411) -> (24.760231, 17.568462)
  line L4 (23.260231, 14.970386) -> (24.760231, 15.836411)
  line L5 (21.760231, 15.836411) -> (23.260231, 14.970386)
extrude "Extrusion11" cut sketch "Sketch_3 outline for Extrusion11" along normal mid plane 3
ref_plane "ANBAU_XY" through (45.1, 13.8, 80) normal (0, 0, 1) x (1, 0, 0)
ref_plane "ANBAU_YZ" through (45.1, 13.8, 80) normal (1, 0, 0) x (0, 1, 0)
ref_plane "ANBAU_ZX" through (45.1, 13.8, 80) normal (0, 1, 0) x (0, 0, 1)
ref_plane "CSL_2_1_XY" through (23.5, 35, 15.8) normal (0, -1, 0) x (1, 0, 0)
ref_plane "CSL_2_1_YZ" through (23.5, 35, 15.8) normal (1, 0, 0) x (0, 0, 1)
ref_plane "CSL_2_1_ZX" through (23.5, 35, 15.8) normal (0, 0, 1) x (0, -1, 0)
ref_plane "CSL_2_2_XY" through (23.5, 35, 25.8) normal (0, -1, 0) x (1, 0, 0)
ref_plane "CSL_2_2_YZ" through (23.5, 35, 25.8) normal (1, 0, 0) x (0, 0, 1)
ref_plane "CSL_2_2_ZX" through (23.5, 35, 25.8) normal (0, 0, 1) x (0, -1, 0)
ref_plane "CSL_3_1_XY" through (13.5, 17.1, 0) normal (0, 0, 1) x (1, 0, 0)
ref_plane "CSL_3_1_YZ" through (13.5, 17.1, 0) normal (1, 0, 0) x (0, 1, 0)
ref_plane "CSL_3_1_ZX" through (13.5, 17.1, 0) normal (0, 1, 0) x (0, 0, 1)
ref_plane "CSL_3_2_XY" through (33.5, 17.1, 0) normal (0, 0, 1) x (1, 0, 0)
ref_plane "CSL_3_2_YZ" through (33.5, 17.1, 0) normal (1, 0, 0) x (0, 1, 0)
ref_plane "CSL_3_2_ZX" through (33.5, 17.1, 0) normal (0, 1, 0) x (0, 0, 1)
ref_plane "DIM_YOKE_NULL_XY" through (0, 0, 0) normal (0, 0, 1) x (1, 0, 0)
ref_plane "DIM_YOKE_NULL_YZ" through (0, 0, 0) normal (1, 0, 0) x (0, 1, 0)
ref_plane "DIM_YOKE_NULL_ZX" through (0, 0, 0) normal (0, 1, 0) x (0, 0, 1)
ref_plane "FDT_DADP1_XY" through (23.5, 35, 15.8) normal (0, 1, 0) x (1, 0, 0)
ref_plane "FDT_DADP1_YZ" through (23.5, 35, 15.8) normal (1, 0, 0) x (0, 0, -1)
ref_plane "FDT_DADP1_ZX" through (23.5, 35, 15.8) normal (0, 0, -1) x (0, 1, 0)
ref_plane "FDT_DADP2_XY" through (23.5, 35, 65.8) normal (0, 1, 0) x (1, 0, 0)
ref_plane "FDT_DADP2_YZ" through (23.5, 35, 65.8) normal (1, 0, 0) x (0, 0, -1)
ref_plane "FDT_DADP2_ZX" through (23.5, 35, 65.8) normal (0, 0, -1) x (0, 1, 0)
ref_plane "IP_KS_XY" through (45.1, 13.8, 9.5) normal (0, 0, -1) x (1, 0, 0)
ref_plane "IP_KS_YZ" through (45.1, 13.8, 9.5) normal (1, 0, 0) x (0, -1, 0)
ref_plane "IP_KS_ZX" through (45.1, 13.8, 9.5) normal (0, -1, 0) x (0, 0, -1)
ref_plane "IP_SD_XY" through (14.2, 18.3, 130.6) normal (0, 0, 1) x (1, 0, 0)
ref_plane "IP_SD_YZ" through (14.2, 18.3, 130.6) normal (1, 0, 0) x (0, 1, 0)
ref_plane "IP_SD_ZX" through (14.2, 18.3, 130.6) normal (0, 1, 0) x (0, 0, 1)
body "Solid1"
